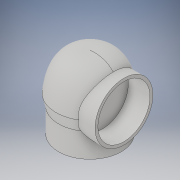
# Autodesk Inventor part: tete2
Saved by Autodesk Inventor 2018 (Build 220112000, 112)
## iProperties
Created: 2018-04-09
Part Number: tete2
Material: Generic
Document SubType Name: Modeling
Designer: usrvauban02
Density: 1 g/cm^3
Appearance: Default
Author: usrvauban02
## iProperties of the stored document Part1_3DPrint.ipt
Created: 2018-04-09
Part Number: Part1_3DPrint
Material: Generic
Document SubType Name: Modeling
Designer: usrvauban02
Density: 1 g/cm^3
Appearance: Default
Author: usrvauban02
Autodesk Inventor part; units mm, degrees
ref_plane "YZ Plane" through (0, 0, 0) normal (1, 0, 0) x (0, 1, 0)
ref_plane "XZ Plane" through (0, 0, 0) normal (0, 1, 0) x (-1, 0, 0)
ref_plane "XY Plane" through (0, 0, 0) normal (0, 0, 1) x (1, 0, 0)
sketch "Sketch1" plane through (0, 0, 0) normal (0, 0, 1) x (1, 0, 0)
  line L0 (0, 0) -> (65, 0)
  line L1 (0, 126.1861) -> (0, 150)
  line L2 (0, 18.2402) -> (0, 0)
  line L3 (0, 126.1861) -> (0, 18.2402)
  line L4 (65, 0) -> (65, 50.0668)
  line L5 (0, 150) -> (62.6016, 156.9829) construction
  line L6 (62.6016, 156.9829) -> (70.4299, 73.1619) construction
  spline S0 degree 2 poles (0, 150) (62.6016, 156.9829) (70.4299, 73.1619) knots 1 1 1 2 2 2
  line L7 (65, 50.0668) -> (70.4299, 73.1619) construction
  spline S1 degree 1 poles (65, 50.0668) (70.4299, 73.1619) knots 1 1 2 2
  point P0 (84.7515, 38.5438)
  dimension "d1" = 65
  dimension "d2" = 150
  constraints: 10 end point, 3 vertical, 1 collinear, 1 horizontal, 6 other
  measures "d1" distance of L0.start L0.end
  measures "d2" distance of L0.start L1.end
revolve "Revolution1" add sketch "Sketch1" angle 360 about axis through (0, 126.1861, 0) along (0, -1, 0)
sketch "Sketch2" plane through (0, 0, 0) normal (1, 0, 0) x (0, 1, 0)
  line L0 (0, 75) -> (0, -75) projected
  circle A0 centre (75, 0) radius 60
  point P0 (0, 0)
  point P1 (150, 0)
  dimension "d4" = 120
  dimension "d25" = 75
  constraints: 1 centre point
  measures "d4" diameter of A0
  measures "d25" distance from line of A0.centre L0
extrude "Extrusion1" add sketch "Sketch2" along normal blind 70.45
hole "Hole1" at (70.45, 75, 0) direction (-1, 0, 0) diameter 108 depth 45
body "Solid1"
